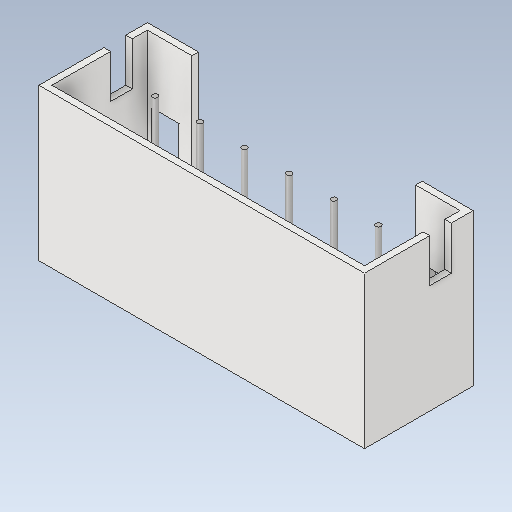
# Autodesk Inventor part: Part6
Saved by Autodesk Inventor 2020 (Build 240168000, 168)
## iProperties
Created: 2020-06-30
Part Number: Part6
Material: Generic
Document SubType Name: Modeling
Designer: IVAN
Density: 1 g/cm^3
Appearance: Default
Author: IVAN
Autodesk Inventor part; units mm, degrees
ref_plane "YZ Plane" through (0, 0, 0) normal (1, 0, 0) x (0, 1, 0)
ref_plane "XZ Plane" through (0, 0, 0) normal (0, 1, 0) x (-1, 0, 0)
ref_plane "XY Plane" through (0, 0, 0) normal (0, 0, 1) x (1, 0, 0)
sketch "Sketch1" plane through (0, 0, 0) normal (0, 1, 0) x (-1, 0, 0)
  line L0 (-7.5, -2.5) -> (7.5, -2.5)
  line L1 (7.5, -2.5) -> (7.5, 2.5)
  line L2 (7.5, 2.5) -> (-7.5, 2.5)
  line L3 (-7.5, 2.5) -> (-7.5, -2.5)
  line L4 (-7.5, -2.5) -> (7.5, 2.5) construction
  line L5 (7.5, -2.5) -> (-7.5, 2.5) construction
  point P0 (0, 0)
  dimension "d0" = 15
  dimension "d1" = 5
  constraints: 12 end point, 2 midpoint, 2 parallel, 1 horizontal, 1 perpendicular
  measures "d0" distance of L2.end L1.end
  measures "d1" distance of L1.end L0.end
extrude "Extrusion1" add sketch "Sketch1" along normal blind 1
sketch "Sketch2" plane through (0, 1, 0) normal (0, 1, 0) x (1, 0, 0)
  line L0 (7.5, 2.5) -> (-7.5, 2.5) projected
  line L1 (-7.5, 2.5) -> (-7.5, -2.5) projected
  line L2 (-7.5, -2.5) -> (7.5, -2.5) projected
  line L3 (7.5, -2.5) -> (7.5, 2.5) projected
  line L4 (-5.1536, 2.5) -> (-5.1536, 2.2)
  line L5 (-5.1536, 2.2) -> (-7.2, 2.2)
  line L6 (-7.2, 2.2) -> (-7.2, -2.2)
  line L7 (-7.2, -2.2) -> (0, -2.2)
  line L8 (0, -2.2) -> (0, -2.5)
  line L9 (7.5, 2.5) -> (-7.5, 2.5) projected
  line L10 (-5.1536, 2.5) -> (-7.5, 2.5)
  line L11 (-7.5, 2.5) -> (-7.5, -2.5)
  point P0 (0, 0)
  dimension "d4" = 0.3
  dimension "d5" = 0.3
  dimension "d6" = 0.3
  constraints: 14 end point, 4 perpendicular, 1 horizontal, 1 midpoint, 1 point on line, 1 vertical
  measures "d4" distance of L4.start L4.end
  measures "d5" distance between parallel lines of L2 L7
  measures "d6" distance between parallel lines of L1 L6
extrude "Extrusion2" add sketch "Sketch2" along normal blind 6 contours L4 L5 L6 L7 L8 L2 L1 L0
mirror "Mirror1" about plane through (0, 0, 0) normal (1, 0, 0) of "Extrusion2"
sketch "Sketch3" plane through (7.5, 0, -2.5) normal (0, 0, -1) x (-1, 0, 0)
  line L0 (0, 0) -> (15, 0) projected
  line L1 (15, 0) -> (15, 7) projected
  line L2 (12.6536, 7) -> (15, 7) projected
  line L3 (12.6536, 1) -> (12.6536, 7) projected
  line L4 (2.3464, 1) -> (12.6536, 1) projected
  line L5 (2.3464, 1) -> (2.3464, 7) projected
  line L6 (2.3464, 7) -> (0, 7) projected
  line L7 (0, 0) -> (0, 7) projected
  line L8 (14.5, 1.5) -> (13.25, 1.5)
  line L9 (13.25, 1.5) -> (13.25, 4)
  line L10 (13.25, 4) -> (14.5, 4)
  line L11 (14.5, 4) -> (14.5, 1.5)
  line L12 (14.5, 1.5) -> (13.25, 4) construction
  line L13 (13.25, 1.5) -> (14.5, 4) construction
  point P0 (7.5, 0)
  point P1 (13.875, 2.75)
  dimension "d9" = 1.25
  dimension "d10" = 2.5
  dimension "d11" = 0.5
  dimension "d12" = 0.5
  constraints: 12 end point, 2 midpoint, 2 parallel, 1 horizontal, 1 perpendicular
  measures "d9" distance of L8.start L8.end
  measures "d10" distance of L10.end L8.start
  measures "d11" distance between parallel lines of L1 L11
  measures "d12" distance between parallel lines of L4 L8
extrude "Extrusion3" cut sketch "Sketch3" against normal up to surface (0.3 mm away) contours L8 L9 L10 L11
mirror "Mirror2" about plane through (0, 0, 0) normal (1, 0, 0) of "Extrusion3"
sketch "Sketch4" plane through (0, 1, 0) normal (0, 1, 0) x (1, 0, 0)
  line L0 (0, 0) -> (-21.8742, 0)
  circle A0 centre (-5.1429, 0.5) radius 0.125
  line L1 (7.2, -2.2) -> (7.2, 2.2) projected
  line L2 (-7.2, -2.2) -> (-7.2, 2.2) projected
  dimension "d15" = 0.25
  dimension "d16" = 0.5
  dimension "d17" = 14.4
  dimension "d18" = 2.0571
  constraints: 2 end point, 1 centre point, 1 horizontal
  measures "d15" diameter of A0
  measures "d16" distance from line of L0 A0.centre
  measures "d17" distance between parallel lines of L1 L2
  measures "d18" distance from line of L2 A0.centre
extrude "Extrusion4" add sketch "Sketch4" along normal blind 5.25 and the other way blind 2.625
pattern_linear "Rectangular Pattern1" count 6 spacing 2.0571 along (1, 0, 0) of "Extrusion4"
sketch "Sketch5" plane through (-7.5, 0, -2.5) normal (-1, 0, 0) x (0, 0, 1)
  line L0 (0, 0) -> (5, 0) projected
  line L1 (5, 0) -> (5, 7) projected
  line L2 (0, 7) -> (5, 7) projected
  line L3 (0, 0) -> (0, 7) projected
  line L4 (1, 7) -> (2, 7)
  line L5 (2, 7) -> (2, 5)
  line L6 (2, 5) -> (1, 5)
  line L7 (1, 5) -> (1, 7)
  point P0 (2.5, 0)
  dimension "d26" = 1
  dimension "d27" = 2
  dimension "d28" = 1
  constraints: 8 end point, 2 parallel, 1 horizontal, 1 perpendicular, 1 point on line
  measures "d26" distance of L5.end L6.end
  measures "d27" distance of L4.end L5.end
  measures "d28" distance between parallel lines of L3 L7
extrude "Extrusion5" cut sketch "Sketch5" against normal up to surface (0.3 mm away) contours L2 L5 L6 L7
mirror "Mirror3" about plane through (0, 0, 0) normal (1, 0, 0) of "Extrusion5"
equation "\"d5\" = d4"
equation "\"d6\" = d5"
equation "\"d12\" = d11"
equation "\"d18\" = 0.142857 * d17"
equation "\"d23\" = 0.142857 * d17"
equation "\"d28\" = d26"
body "Solid1"
